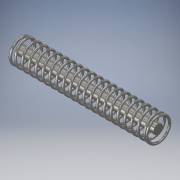
# Autodesk Inventor part: BT504_trajan20_21
Saved by Autodesk Inventor 2022.2 (Build 262287000, 287)
## iProperties
Company: HTBLA Kaindorf
RuleStatus: InUse
Created: 2022-08-19
Part Number: BT504_trajan20_21
Project: Zeichenmaschine_v2
Material: Stahl, Legierung
Description: Stifthalter_feder
Document SubType Name: Modeling
Designer: trajan20
Density: 7.73 g/cm^3
Appearance: Halbpoliert
Mass: 1.24827 g
Surface Area: 7.29347 cm^2
Volume: 0.161484 cm^3
AfterDocNew0: iProperties-Editor_aufrufen
Author: jan
Keywords: 2021
Autodesk Inventor part; units mm, degrees
ref_plane "YZ Plane" through (0, 0, 0) normal (1, 0, 0) x (0, 1, 0)
ref_plane "XZ Plane" through (0, 0, 0) normal (0, 1, 0) x (-1, 0, 0)
ref_plane "XY Plane" through (0, 0, 0) normal (0, 0, 1) x (1, 0, 0)
sketch "Skizze3" plane through (0, 0, 0) normal (1, 0, 0) x (0, 1, 0)
  point P0 (0, 0)
sketch "Skizze5" plane through (0, 0, 0) normal (0, 1, 0) x (-1, 0, 0)
  circle A0 centre (0, 0) radius 2.5
  dimension "d16" = 5
  constraints: 1 centre point, 1 coincident
  measures "d16" diameter of A0
ref_plane "Arbeitsebene2" through (0, 30, 0) normal (0, 1, 0) x (-1, 0, 0)
sketch "Skizze6" plane through (0, 30, 0) normal (0, 1, 0) x (-1, 0, 0)
  circle A0 centre (0, 0) radius 2.5
  circle A1 centre (0, 0) radius 1
  dimension "d17" = 5
  dimension "d26" = 2
  constraints: 2 centre point, 2 coincident
  measures "d17" diameter of A0
  measures "d26" diameter of A1
ref_plane "Arbeitsebene3" through (0, 0, -2.5) normal (-0.9954715, 0.0950605, 0) x (-0.0950605, -0.9954715, 0)
sketch "Skizze7" plane through (0, 0, -2.5) normal (-0.9954715, 0.0950605, 0) x (-0.0950605, -0.9954715, 0)
  circle A0 centre (0, 0) radius 0.25
  point P0 (0, 2.5)
  dimension "d18" = 0.5
  constraints: 1 centre point
  measures "d18" diameter of A0
sketch3d "3D-Skizze2"
  helix H0 starts at (0, 0, -2.5) axis through (0, 0, 0) along (0, 1, 0) pitch 1.5 turns 20 hand right
sweep "Sweeping2" add profiles "Skizze7" path "3D-Skizze2"
sweep "Sweeping3" add profiles "Skizze7" path "Skizze5"
sketch "Skizze8" plane through (0, 30.0001, -2.4999) normal (-0.9954715, 0.0950605, 0) x (0, 0, 1)
  circle A0 centre (0, 0) radius 0.25
  point P0 (2.4999, -29.8643)
  dimension "d23" = 0.5
  constraints: 1 centre point
  measures "d23" diameter of A0
sweep "Sweeping4" add profiles "Skizze8" path "Skizze6" path curves A0
sketch "Skizze9" plane through (0, 0, 0) normal (0, 0, 1) x (1, 0, 0)
  point P0 (0, 0)
extrude "Extrusion3" add sketch "Skizze6" against normal blind 30 contours A1
